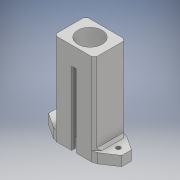
# Autodesk Inventor part: RescueKit-Pipev2
Saved by Autodesk Inventor 2018.3 (Build 223284000, 284)
## iProperties
Created: 2019-03-13
Part Number: RescueKit-Pipev2
Material: 一般
Document SubType Name: Modeling
Designer: shun2
Density: 1 g/cm^3
Appearance: 既定
Author: shun2
Autodesk Inventor part; units mm, degrees
ref_plane "YZ Plane" through (0, 0, 0) normal (1, 0, 0) x (0, 1, 0)
ref_plane "XZ Plane" through (0, 0, 0) normal (0, 1, 0) x (-1, 0, 0)
ref_plane "XY Plane" through (0, 0, 0) normal (0, 0, 1) x (1, 0, 0)
sketch "スケッチ1" plane through (0, 0, 0) normal (0, 0, 1) x (1, 0, 0)
  line L0 (-16.5, 13) -> (16.5, 13)
  line L1 (16.5, 13) -> (16.5, -13)
  line L2 (16.5, -13) -> (-16.5, -13)
  line L3 (-16.5, -13) -> (-16.5, 13)
  line L4 (-16.5, 13) -> (16.5, -13) construction
  line L5 (16.5, 13) -> (-16.5, -13) construction
  circle A0 centre (0, 0) radius 10
  dimension "d0" = 33
  dimension "d1" = 26
  dimension "d2" = 20
  constraints: 12 end point, 2 midpoint, 2 parallel, 1 centre point, 1 coincident, 1 horizontal, 1 perpendicular
  measures "d0" distance of L1.end L2.end
  measures "d1" distance of L0.end L1.end
  measures "d2" diameter of A0
extrude "押し出し1" add sketch "スケッチ1" along normal blind 70
sketch "スケッチ2" plane through (-16.5, -13, 0) normal (0, -1, 0) x (1, 0, 0)
  line L0 (18.5, 60) -> (18.5, 0)
  line L1 (18.5, 0) -> (14.5, 0)
  line L2 (14.5, 0) -> (14.5, 60)
  line L3 (18.5, 70) -> (14.5, 0) construction
  line L4 (18.5, 0) -> (14.5, 70) construction
  line L5 (0, 0) -> (33, 0) projected
  line L6 (18.5, 60) -> (14.5, 60)
  point P0 (16.5, 0)
  point P1 (16.5, 35)
  dimension "d5" = 4
  constraints: 12 end point, 3 perpendicular, 2 midpoint, 1 parallel
  measures "d5" distance of L0.end L1.end
extrude "押し出し2" cut sketch "スケッチ2" against normal blind 50
sketch "スケッチ3" plane through (0, 0, 70) normal (0, 0, 1) x (1, 0, 0)
  line L0 (-16.5, -13) -> (16.5, -13) projected
  line L1 (16.5, -13) -> (16.5, 13) projected
  line L2 (16.5, 13) -> (-16.5, 13) projected
  circle A0 centre (0, 0) radius 10 projected
  circle A1 centre (0, 0) radius 10 projected
  line L3 (16.5, 13) -> (-16.5, 13) projected
  line L4 (-16.5, 13) -> (-16.5, -13) projected
  line L5 (-16.5, -13) -> (16.5, -13) projected
  line L6 (16.5, -13) -> (-16.5, -13)
  line L7 (-16.5, -13) -> (-16.5, 13)
  line L8 (-16.5, 13) -> (16.5, 13)
  line L9 (16.5, 13) -> (16.5, -13)
  circle A2 centre (0, 0) radius 10
  line L10 (16.5, -13) -> (16.5, 13) projected
  line L11 (-16.5, 13) -> (-16.5, -13) projected
  dimension "d8" = 20
  constraints: 8 end point, 2 parallel, 1 centre point, 1 coincident, 1 horizontal, 1 perpendicular
  measures "d8" diameter of A2
extrude "押し出し3" add sketch "スケッチ3" along normal blind 5
sketch "スケッチ4" plane through (0, 0, 0) normal (0, 0, -1) x (-1, 0, 0)
  line L0 (30, -4) -> (30, 4)
  line L1 (-30, 4) -> (-30, -4)
  line L2 (-30, -4) -> (30, 4) construction
  line L3 (30, -4) -> (-30, 4) construction
  line L4 (-2, 13) -> (-16.5, 13) projected
  line L5 (-16.5, 13) -> (-30, 4)
  line L6 (-16.5, 13) -> (-16.5, -13) projected
  line L7 (-30, -4) -> (-16.5, -13)
  line L8 (2, -9.798) -> (2, -13) projected
  line L9 (2, -13) -> (16.5, -13) projected
  line L10 (16.5, -13) -> (16.5, 13) projected
  line L11 (16.5, 13) -> (2, 13) projected
  line L12 (2, 13) -> (2, 9.798) projected
  arc A0 (2, -9.798) -> (2, 9.798) centre (0, 0) ccw projected
  line L13 (-2, -13) -> (-2, -9.798) projected
  arc A1 (-2, 9.798) -> (-2, -9.798) centre (0, 0) ccw projected
  line L14 (-2, 9.798) -> (-2, 13) projected
  line L15 (-2, 13) -> (-16.5, 13) projected
  line L16 (-16.5, 13) -> (-16.5, -13) projected
  line L17 (-16.5, -13) -> (-2, -13) projected
  line L18 (16.5, -13) -> (30, -4)
  line L19 (30, 4) -> (16.5, 13)
  circle A2 centre (-23.25, 0) radius 1.75
  circle A3 centre (23.25, 0) radius 1.75
  dimension "d15" = 3.5
  dimension "d16" = 3.5
  constraints: 16 end point, 2 centre point, 2 midpoint, 1 parallel
  measures "d15" diameter of A2
  measures "d16" diameter of A3
extrude "押し出し4" add sketch "スケッチ4" against normal blind 8 contours L18 L10 L19 L0 | L5 L6 L7 L1
chamfer "面取り1" distance 2 angle 45 10 edges at (16.5, 0, 8) (-16.5, 0, 8) (16.5, -13, 41.5) (16.5, 13, 41.5) (-16.5, -13, 41.5) (-16.5, -13, 4) (16.5, -13, 4) (-16.5, 13, 41.5) (-16.5, 13, 4) (16.5, 13, 4)
